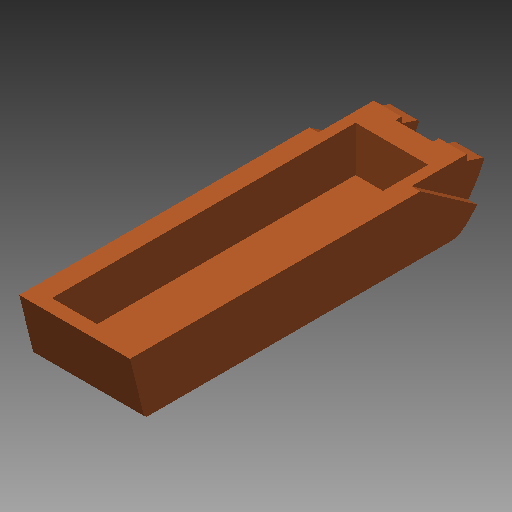
# Autodesk Inventor part: CH20M LF OR 1103640000
Saved by Autodesk Inventor 2019.3 (Build 233278000, 278)
## iProperties
Category: PARTsolutions
Company: WEIDMUELLER
Created: 2018-11-15
Part Number: CH20M LF OR 1103640000
Material: Generic
Catalog Web Link: www.cadenas.de
Description: CH20M LF-CH20M
Vendor: WEIDMUELLER
Document SubType Name: Modeling
Designer: psadmin
Manufacturer: WEIDMUELLER
Mass: 1.70685 g
Surface Area: 20.492 cm^2
Volume: 1.70685 cm^3
Density: 1 g/cm^3
Appearance: PSOLRGB-219-112-51
PSOL_IDENT_0: {$CADENAS_DATA\23d-libs\weidmueller\elektronikgehaeuse\einbaugehaeuse\ch20m\einzelteile\ch20m22-5\ch
PSOL_IDENT_1: 20m-lf.prj},186 {VTYP=3D},{NB=CH20M LF OR 1103640000},{LINA=CH20M LF OR 1103640000},{NN=CH20M LF},{D
PSOL_IDENT_2: ATE=18.01.2013 16:41:05},{GEOMDATE=28.10.2012 09:24:00},{VERSION=},{LINEID=20},{WBVAR=},{WBNUMERIC=}
PSOL_IDENT_3: {NB=CH20M LF OR 1103640000},{LINA=CH20M LF OR 1103640000},{KT=DUMMY},{BEST=1103640000},{BZ=CH20M L
PSOL_IDENT_4: F OR},{AB=Rastfuss},{F=orange},{FCODE=0.86,0.44,0.20,0.00}
NN: CH20M LF
NT: CH20M
NB: CH20M LF OR 1103640000
NBSYN: $BZ. $BEST.
LINA: CH20M LF OR 1103640000
BEST: 1103640000
BZ: CH20M LF OR
AB: Locking foot
F: orange
SUPPLIER: WEIDMUELLER
ARTICLENO: CH20M LF OR 1103640000
BOMINFO: CH20M LF OR 1103640000
CREATOR: CADENAS GmbH
Title: CH20M LF OR 1103640000
Author: Cadenas PARTsolutions
Comments: CH20M
Autodesk Inventor part; units mm, degrees
sketch "Sketch_1" plane through (0, 0, 0) normal (1, 0, 0) x (0, 1, 0)
  line L0 (6.6, 0) -> (0.379, -1.5511)
  arc A0 (0.379, -1.5511) -> (0, -2.0362) centre (0.5, -2.0362) ccw
  line L1 (0, -2.0362) -> (0, -36.1119)
  arc A1 (0, -36.1119) -> (0.6316, -37.7729) centre (2.5, -36.1119) ccw
  arc A2 (0.6316, -37.7729) -> (5.0923, -40.9212) centre (9.6, -29.8) ccw
  arc A3 (5.0923, -40.9212) -> (5.3576, -40.7976) centre (5.1674, -40.7358) ccw
  line L2 (5.3576, -40.7976) -> (5.9417, -39)
  line L3 (5.9417, -39) -> (6.6, -39)
  line L4 (6.6, -39) -> (6.6, 0)
  constraints: 10 end point, 8 point on circle, 4 centre point
extrude "Extrusion1" add sketch "Sketch_1" along normal mid plane 12.5
sketch "Sketch_2" plane through (0, 0, 0) normal (1, 0, 0) x (0, 1, 0)
  line L0 (6.6, -1.5459) -> (1.879, -2.723)
  arc A0 (1.879, -2.723) -> (1.5, -3.2081) centre (2, -3.2081) ccw
  line L1 (1.5, -3.2081) -> (1.5, -35.8)
  line L2 (1.5, -35.8) -> (6.6, -35.8)
  line L3 (6.6, -35.8) -> (6.6, -1.5459)
  constraints: 8 end point, 2 point on circle, 1 centre point
extrude "Extrusion2" cut sketch "Sketch_2" along normal mid plane 8.2
sketch "Sketch_3" plane through (6.25, 0, 0) normal (1, 0, 0) x (0, 0, -1)
  line L0 (32.75, 6.6) -> (42, 0.1231)
  line L1 (42, 0.1231) -> (42, 6.6)
  line L2 (42, 6.6) -> (32.75, 6.6)
  constraints: 6 end point
extrude "Extrusion3" cut sketch "Sketch_3" against normal blind 1
sketch "Sketch_4" plane through (-6.25, 0, 0) normal (1, 0, 0) x (0, 0, -1)
  line L0 (32.75, 6.6) -> (42, 0.1231)
  line L1 (42, 0.1231) -> (42, 6.6)
  line L2 (42, 6.6) -> (32.75, 6.6)
  constraints: 6 end point
extrude "Extrusion4" cut sketch "Sketch_4" along normal blind 1
sketch "Sketch_5" plane through (0, 0, 0) normal (1, 0, 0) x (0, 1, 0)
  line L0 (6.6, -38.32) -> (0, -38.32)
  line L1 (0, -38.32) -> (0, -42)
  line L2 (0, -42) -> (6.6, -42)
  line L3 (6.6, -42) -> (6.6, -38.32)
  constraints: 8 end point
extrude "Extrusion5" cut sketch "Sketch_5" along normal mid plane 4.2
ref_plane "CP_XY" through (0, 6.6, 0) normal (0, 0, 1) x (1, 0, 0)
ref_plane "CP_YZ" through (0, 6.6, 0) normal (1, 0, 0) x (0, 1, 0)
ref_plane "CP_ZX" through (0, 6.6, 0) normal (0, 1, 0) x (0, 0, 1)
body "Solid1"
